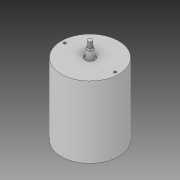
# Autodesk Inventor part: boma_2kw_motor
Saved by Autodesk Inventor 2019 (Build 230136000, 136)
## iProperties
Created: 2018-09-22
Part Number: boma_2kw_motor
Material: Generic
Document SubType Name: Modeling
Designer: Callum Snowden
Mass: 1228.83 g
Surface Area: 655.716 cm^2
Volume: 1228.83 cm^3
Density: 1 g/cm^3
Appearance: Default
Author: Callum Snowden
Autodesk Inventor part; units mm, degrees
ref_plane "YZ Plane" through (0, 0, 0) normal (1, 0, 0) x (0, 1, 0)
ref_plane "XZ Plane" through (0, 0, 0) normal (0, 1, 0) x (-1, 0, 0)
ref_plane "XY Plane" through (0, 0, 0) normal (0, 0, 1) x (1, 0, 0)
sketch "Sketch1" plane through (0, 0, 0) normal (0, 1, 0) x (-1, 0, 0)
  circle A0 centre (0, 0) radius 54
  dimension "d0" = 108
  constraints: 1 centre point, 1 coincident
  measures "d0" diameter of A0
extrude "Extrusion1" add sketch "Sketch1" along normal blind 134
sketch "Sketch2" plane through (0, 134, 0) normal (0, 1, 0) x (1, 0, 0)
  circle A0 centre (0, 0) radius 9
  dimension "d3" = 18
  constraints: 1 centre point, 1 coincident
  measures "d3" diameter of A0
extrude "Extrusion2" cut sketch "Sketch2" against normal blind 2.5
sketch "Sketch3" plane through (0, 131.5, 0) normal (0, 1, 0) x (1, 0, 0)
  circle A0 centre (0, 0) radius 6
  dimension "d6" = 12
  constraints: 1 centre point, 1 coincident
  measures "d6" diameter of A0
extrude "Extrusion3" add sketch "Sketch3" along normal blind 17
sketch "Sketch4" plane through (0, 148.5, 0) normal (0, 1, 0) x (1, 0, 0)
  line L0 (-4.25, -2.6339) -> (-4.25, 2.6339)
  line L1 (4.25, -2.6339) -> (4.25, 2.6339)
  arc A0 (-4.25, -2.6339) -> (4.25, -2.6339) centre (0, 0) ccw
  arc A1 (4.25, 2.6339) -> (-4.25, 2.6339) centre (0, 0) ccw
  dimension "d10" = 8.5
  constraints: 4 end point, 4 point on circle, 2 centre point, 1 coincident, 1 parallel, 1 vertical
  measures "d10" distance between parallel lines of L1 L0
extrude "Extrusion4" add sketch "Sketch4" along normal blind 3.5
sketch "Sketch5" plane through (0, 134, 0) normal (0, 1, 0) x (1, 0, 0)
  line L0 (75.6, 0) -> (-75.6, 0) construction
  line L1 (0, 75.6) -> (0, -75.6) construction
  point P0 (0, 0)
  point P1 (-47.25, 0)
  point P2 (47.25, 0)
  dimension "d16" = 94.5
  constraints: 2 point on line, 1 symmetric about line
  measures "d16" distance of point (-47.25, 0) point (47.25, 0)
hole "Hole1" at (-47.25, 134, 0) at (47.25, 134, 0) direction (0, -1, 0) diameter 4.917 depth 10 tip angle 118 thread size "M6x1" class "6H" standard "ISO Metric profile"
sketch "Sketch6" plane through (0, 0, 0) normal (0, -1, 0) x (1, 0, 0)
  circle A0 centre (47.25, 0) radius 2.4585
  circle A1 centre (-47.25, 0) radius 2.4585
  line L0 (0, 75.6) -> (0, -75.6) construction
  point P0 (0, 0)
  dimension "d24" = 94.5
  constraints: 2 centre point, 1 symmetric about line
  measures "d24" distance of A1.centre A0.centre
hole "Hole2" at (47.25, 0, 0) at (-47.25, 0, 0) direction (0, 1, 0) diameter 4.917 depth 10 tip angle 118 thread size "M6x1" class "6H" standard "ISO Metric profile"
sketch "Sketch7" plane through (0, 152, 0) normal (0, 1, 0) x (1, 0, 0)
  circle A0 centre (0, 0) radius 4
  dimension "d32" = 8
  constraints: 1 centre point, 1 coincident
  measures "d32" diameter of A0
extrude "Extrusion5" add sketch "Sketch7" along normal blind 10.5
thread "Thread1" size "M8x1.25" class "6g" standard "ISO Metric profile" full length
body "Solid1"
